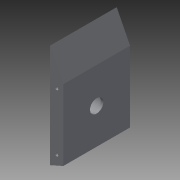
# Autodesk Inventor part: bocnice_kratsi
Saved by Autodesk Inventor 2015 (Build 190159000, 159)
## iProperties
Created: 2015-01-01
Part Number: bocnice_kratsi
Material: Generic
Document SubType Name: Modeling
Designer: Turboslimak
Density: 1 g/cm^3
Appearance: Default
Author: Turboslimak
Autodesk Inventor part; units mm, degrees
ref_plane "YZ Plane" through (0, 0, 0) normal (1, 0, 0) x (0, 1, 0)
ref_plane "XZ Plane" through (0, 0, 0) normal (0, 1, 0) x (-1, 0, 0)
ref_plane "XY Plane" through (0, 0, 0) normal (0, 0, 1) x (1, 0, 0)
sketch "Sketch1" plane through (0, 0, 0) normal (0, 1, 0) x (-1, 0, 0)
  line L0 (-5, 26.5) -> (5, 26.5)
  line L1 (5, 26.5) -> (5, -26.5)
  line L2 (5, -26.5) -> (-5, -26.5)
  line L3 (-5, -26.5) -> (-5, 26.5)
  line L4 (5, -26.5) -> (5, -30.9444)
  line L5 (5, -30.9444) -> (-5, -26.5)
  line L6 (5, -30.9444) -> (5, 46.5)
  line L7 (5, 46.5) -> (-5, 26.5)
  line L8 (-5, -26.5) -> (0, -26.5)
  line L9 (-5, -21.5) -> (-5, -26.5)
  line L10 (5, 26.5) -> (0, 26.5)
  line L11 (5, 21.5) -> (5, 26.5)
  circle A0 centre (0, 21.5) radius 1.25
  circle A1 centre (0, -21.5) radius 1.25
  point P0 (0, 0)
  dimension "d0" = 10
  dimension "d1" = 53
  dimension "d2" = 4.4444
  dimension "d3" = 77.4444
  dimension "d8" = 2.5
  dimension "d9" = 2.5
  constraints: 24 end point, 3 horizontal, 3 parallel, 2 centre point, 1 perpendicular, 1 point on line
  measures "d0" distance of L1.end L2.end
  measures "d1" distance of L0.end L1.end
  measures "d2" distance of L1.end L4.end
  measures "d3" distance of L4.end L6.end
  measures "d8" diameter of A0
  measures "d9" diameter of A1
extrude "Extrusion1" add sketch "Sketch1" along normal blind 50
sketch "Sketch2" plane through (5, 0, 26.5) normal (1, 0, 0) x (0, 0, -1)
  line L0 (53, 0) -> (0, 0)
  line L1 (0, 0) -> (0, 50)
  line L2 (0, 50) -> (53, 50)
  line L3 (53, 50) -> (53, 0)
  line L4 (26.5, 0) -> (26.5, 25)
  circle A0 centre (26.5, 25) radius 7.5
  circle A1 centre (26.5, 25) radius 5
  dimension "d12" = 25
  dimension "d13" = 15
  dimension "d16" = 10
  constraints: 10 end point, 2 centre point, 2 coincident, 2 parallel, 1 horizontal, 1 perpendicular, 1 vertical
  measures "d12" distance of L4.start L4.end
  measures "d13" diameter of A0
  measures "d16" diameter of A1
extrude "Extrusion2" cut sketch "Sketch2" against normal blind 10 contours A1 | A0
extrude "Extrusion3" add sketch "Sketch2" against normal blind 2 contours A0
body "Solid1"
